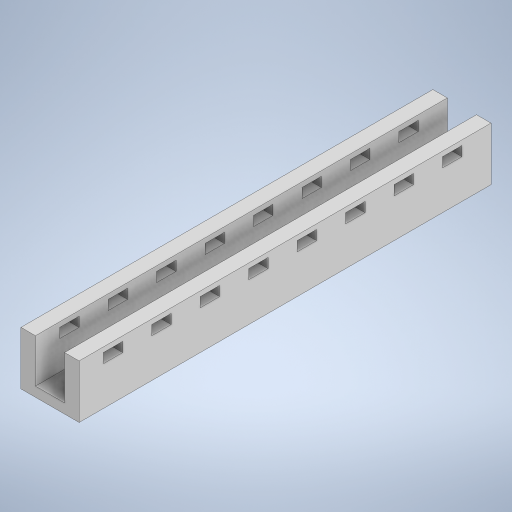
# Autodesk Inventor part: рейка кати
Saved by Autodesk Inventor 2024.2 (Build 282272000, 272)
## iProperties
Created: 2026-01-09
Part Number: рейка кати
Material: Типовые
Document SubType Name: Modeling
Designer: Service
Density: 1 g/cm^3
Appearance: По умолчанию
Author: Service
Autodesk Inventor part; units mm, degrees
ref_plane "YZ Plane" through (0, 0, 0) normal (1, 0, 0) x (0, 1, 0)
ref_plane "XZ Plane" through (0, 0, 0) normal (0, 1, 0) x (-1, 0, 0)
ref_plane "XY Plane" through (0, 0, 0) normal (0, 0, 1) x (1, 0, 0)
sketch "Эскиз1" plane through (0, 0, 0) normal (0, 1, 0) x (-1, 0, 0)
  line L0 (-6, -42.5) -> (6, -42.5)
  line L1 (6, -42.5) -> (6, 42.5)
  line L2 (6, 42.5) -> (-6, 42.5)
  line L3 (-6, 42.5) -> (-6, -42.5)
  line L4 (-6, -42.5) -> (6, 42.5) construction
  line L5 (6, -42.5) -> (-6, 42.5) construction
  circle A0 centre (0, 0) radius 2
  circle A1 centre (0, 22) radius 2.1514
  circle A2 centre (0, -22) radius 2
  dimension "d0" = 4
  dimension "d1" = 22
  dimension "d2" = 22
  dimension "d3" = 85
  dimension "d4" = 12
  constraints: 12 end point, 3 centre point, 2 midpoint, 2 parallel, 1 coincident, 1 equal radius, 1 horizontal, 1 perpendicular
  measures "d0" diameter of A0
  measures "d1" distance of A1.centre point (0, 0)
  measures "d2" distance of A2.centre point (0, 0)
  measures "d3" distance of L0.end L1.end
  measures "d4" distance of L1.end L2.end
extrude "Выдавливание1" add sketch "Эскиз1" along normal blind 2
sketch "Эскиз2" plane through (0, 2, 0) normal (0, 1, 0) x (1, 0, 0)
  line L0 (-6, 42.5) -> (-6, -42.5) projected
  line L1 (-6, -42.5) -> (6, -42.5) projected
  line L2 (6, -42.5) -> (6, 42.5) projected
  line L3 (6, 42.5) -> (-6, 42.5) projected
  circle A0 centre (0, 0) radius 2 projected
  circle A1 centre (0, -22) radius 2.1514 projected
  circle A2 centre (0, 22) radius 2 projected
  line L4 (-6, -42.5) -> (-3, -42.5)
  line L5 (-3, -42.5) -> (-3, 42.5)
  line L6 (-3, 42.5) -> (-6, 42.5)
  line L7 (-6, 42.5) -> (-6, -42.5)
  line L8 (6, 42.5) -> (3, 42.5)
  line L9 (3, 42.5) -> (3, -42.5)
  line L10 (3, -42.5) -> (6, -42.5)
  line L11 (6, -42.5) -> (6, 42.5)
  dimension "d7" = 3
  dimension "d8" = 3
  constraints: 16 end point, 4 parallel, 2 horizontal, 2 perpendicular, 2 point on line
  measures "d7" distance of L4.end L0.end
  measures "d8" distance of L1.end L9.end
extrude "Выдавливание2" add sketch "Эскиз2" along normal blind 9 contours L3 L5 L1 L0 | L3 L2 L1 L9
chamfer "Фаска1" distance 0.5 angle 45 1 edges at (2.1514, 2, 22)
chamfer "Фаска2" distance 0.5 angle 45 2 edges at (2, 2, 0) (2, 2, -22)
sketch "Эскиз3" plane through (6, 0, 42.5) normal (1, 0, 0) x (0, 0, -1)
  line L0 (5, 10) -> (9, 10)
  line L1 (9, 10) -> (9, 8)
  line L2 (9, 8) -> (5, 8)
  line L3 (5, 8) -> (5, 10)
  line L4 (0, 11) -> (85, 11) projected
  line L5 (0, 0) -> (0, 11) projected
  line L6 (15, 10) -> (19, 10)
  line L7 (19, 10) -> (19, 8)
  line L8 (19, 8) -> (15, 8)
  line L9 (15, 8) -> (15, 10)
  line L10 (25, 10) -> (29, 10)
  line L11 (29, 10) -> (29, 8)
  line L12 (29, 8) -> (25, 8)
  line L13 (25, 8) -> (25, 10)
  line L14 (35, 10) -> (39, 10)
  line L15 (39, 10) -> (39, 8)
  line L16 (39, 8) -> (35, 8)
  line L17 (35, 8) -> (35, 10)
  line L18 (45, 10) -> (49, 10)
  line L19 (49, 10) -> (49, 8)
  line L20 (49, 8) -> (45, 8)
  line L21 (45, 8) -> (45, 10)
  line L22 (55, 10) -> (59, 10)
  line L23 (59, 10) -> (59, 8)
  line L24 (59, 8) -> (55, 8)
  line L25 (55, 8) -> (55, 10)
  line L26 (65, 10) -> (69, 10)
  line L27 (69, 10) -> (69, 8)
  line L28 (69, 8) -> (65, 8)
  line L29 (65, 8) -> (65, 10)
  line L30 (75, 10) -> (79, 10)
  line L31 (79, 10) -> (79, 8)
  line L32 (79, 8) -> (75, 8)
  line L33 (75, 8) -> (75, 10)
  point P0 (42.5, 0)
  dimension "d17" = 4
  dimension "d18" = 2
  dimension "d19" = 1
  dimension "d20" = 5
  dimension "d23" = 10
  constraints: 64 end point, 2 horizontal, 2 parallel, 1 collinear, 1 perpendicular, 55 other
  measures "d17" distance of L1.end L2.end
  measures "d18" distance of L0.end L1.end
  measures "d19" distance from line of L4 L0.start
  measures "d20" distance between parallel lines of L5 L3
  measures "d23" distance of L0.start L6.start
extrude "Выдавливание3" cut sketch "Эскиз3" against normal up to surface (12 mm away)
